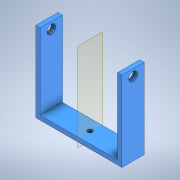
# Autodesk Inventor part: forkV03
Saved by Autodesk Inventor 2021.2 (Build 252289000, 289)
## iProperties
Created: 2020-11-14
Part Number: forkV03
Material: PBT Plastic
Document SubType Name: Modeling
Designer: robst
Density: 1.31 g/cm^3
Appearance: Cyan
Author: robst
Autodesk Inventor part; units mm, degrees
ref_plane "XZ Plane" through (0, 0, 0) normal (0, 1, 0) x (-1, 0, 0)
ref_plane "XY Plane" through (0, 0, 0) normal (0, 0, 1) x (1, 0, 0)
sketch "Sketch1" plane through (0, 0, 0) normal (0, 1, 0) x (-1, 0, 0)
  line L0 (123.19, 31.75) -> (-123.19, 31.75)
  line L1 (-123.19, 31.75) -> (-123.19, -31.75)
  line L2 (-123.19, -31.75) -> (123.19, -31.75)
  line L3 (123.19, -31.75) -> (123.19, 31.75)
  line L4 (123.19, 31.75) -> (-123.19, -31.75) construction
  line L5 (-123.19, 31.75) -> (123.19, -31.75) construction
  point P0 (0, 0)
  dimension "d0" = 246.38
  dimension "d1" = 63.5
  constraints: 12 end point, 2 midpoint, 2 parallel, 1 horizontal, 1 perpendicular
  measures "d0" distance of L0.start L0.end
  measures "d1" distance of L1.end L0.end
extrude "Extrusion1" add sketch "Sketch1" against normal blind 12.7
sketch "Sketch2" plane through (0, 0, 0) normal (0, 1, 0) x (1, 0, 0)
  line L0 (-123.19, -31.75) -> (-123.19, 31.75) projected
  line L1 (-123.19, 31.75) -> (123.19, 31.75) projected
  line L2 (-123.19, -31.75) -> (-110.49, -31.75)
  line L3 (-110.49, -31.75) -> (-110.49, 31.75)
  line L4 (-110.49, 31.75) -> (-123.19, 31.75)
  line L5 (-123.19, 31.75) -> (-123.19, -31.75)
  line L6 (123.19, 31.75) -> (123.19, -31.75) projected
  line L7 (123.19, -31.75) -> (110.49, -31.75)
  line L8 (110.49, -31.75) -> (110.49, 31.75)
  line L9 (110.49, 31.75) -> (123.19, 31.75)
  line L10 (123.19, 31.75) -> (123.19, -31.75)
  point P0 (0, 0)
  dimension "d4" = 12.7
  dimension "d5" = 12.7
  constraints: 16 end point, 4 parallel, 2 horizontal, 2 perpendicular, 2 point on line
  measures "d4" distance between parallel lines of L3 L0
  measures "d5" distance between parallel lines of L6 L8
extrude "Extrusion2" add sketch "Sketch2" along normal blind 215.9
sketch "Sketch3" plane through (-123.19, -12.7, -31.75) normal (-1, 0, 0) x (0, 0, 1)
  line L0 (0, 228.6) -> (63.5, 228.6) construction
  line L1 (31.75, 228.6) -> (31.75, 0) construction
  line L2 (63.5, 0) -> (0, 0) construction
  circle A0 centre (31.75, 209.55) radius 12.7
  line L3 (0, 12.7) -> (0, 228.6) construction
  line L4 (0, 222.25) -> (38.1, 222.25) construction
  point P0 (31.75, 12.7)
  dimension "d8" = 25.4
  dimension "d9" = 6.35
  constraints: 4 end point, 2 midpoint, 2 point on line, 1 centre point, 1 horizontal, 1 tangent
  measures "d8" diameter of A0
  measures "d9" distance between parallel lines of L4 L0
extrude "Extrusion3" cut sketch "Sketch3" against normal through all
sketch "Sketch4" plane through (0, 0, 0) normal (0, 1, 0) x (1, 0, 0)
  line L0 (6.35, 3.6662) -> (6.35, -3.6662)
  line L1 (6.35, -3.6662) -> (0, -7.3323)
  line L2 (0, -7.3323) -> (-6.35, -3.6662)
  line L3 (-6.35, -3.6662) -> (-6.35, 3.6662)
  line L4 (-6.35, 3.6662) -> (0, 7.3323)
  line L5 (0, 7.3323) -> (6.35, 3.6662)
  point P0 (0, 0)
  point P1 (0, 0)
  dimension "d13" = 12.7
  constraints: 12 end point, 1 coincident, 1 vertical, 13 other
  measures "d13" distance between parallel lines of L0 L3
extrude "Extrusion4" cut sketch "Sketch4" against normal through all
body "Solid1"
